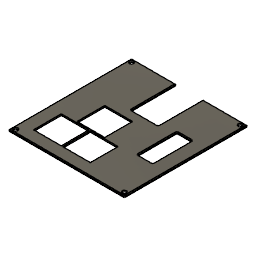
Top (Autodesk Fusion 360 design; units mm, degrees)
part number: 2025-12-11-15-33-41-186
Autodesk Fusion 360 part; units mm, degrees
note: some values were not read from the file. Chosen so that the rebuilt part matches the saved one: a direction; that a step has no effect; which face or edge a step refers to. Set by a fixed rule: which sketch regions a step uses.
sketch "plate-2025-12-11T14_40_51.643Z" plane through (0, 0, 0) normal (0, 0, 1) x (1, 0, 0)
  line L0 (69.2455, 32.444) -> (-10.7545, 32.444)
  line L1 (-10.7545, 32.444) -> (-10.7545, -52.556)
  line L2 (-10.7545, -52.556) -> (69.2455, -52.556)
  line L3 (69.2455, -52.556) -> (69.2455, 32.444)
  line L4 (10.79, 32.444) -> (29.29, 32.444)
  line L5 (64.2455, 27.444) -> (-5.7545, 27.444)
  line L6 (-5.7545, 27.444) -> (-5.7545, -47.556)
  line L7 (-5.7545, -47.556) -> (64.2455, -47.556)
  line L8 (64.2455, -47.556) -> (64.2455, 27.444)
  line L9 (20.04, 63.444) -> (38.54, 63.444)
  line L10 (38.54, 63.444) -> (38.54, 1.444)
  line L11 (38.54, 1.444) -> (20.04, 1.444)
  line L12 (20.04, 1.444) -> (20.04, 63.444)
  circle A0 centre (-8.2545, 29.944) radius 1.45
  circle A1 centre (-8.2545, -50.056) radius 1.45
  circle A2 centre (66.7455, -50.056) radius 1.45
  circle A3 centre (66.7455, 29.944) radius 1.45
  line L13 (8.3105, -5.141) -> (27.3605, -5.141)
  line L14 (27.3605, -5.141) -> (27.3605, -24.191)
  line L15 (27.3605, -24.191) -> (8.3105, -24.191)
  line L16 (8.3105, -24.191) -> (8.3105, -5.141)
  line L17 (18.3405, -25.141) -> (37.3905, -25.141)
  line L18 (37.3905, -25.141) -> (37.3905, -44.191)
  line L19 (37.3905, -44.191) -> (18.3405, -44.191)
  line L20 (18.3405, -44.191) -> (18.3405, -25.141)
  line L21 (-1.7295, -25.146) -> (17.3205, -25.146)
  line L22 (17.3205, -25.146) -> (17.3205, -44.196)
  line L23 (17.3205, -44.196) -> (-1.7295, -44.196)
  line L24 (-1.7295, -44.196) -> (-1.7295, -25.146)
  point P0 (29.29, 32.444)
  dimension "d1" = 80
  dimension "d2" = 85
  dimension "d44" = 75
  dimension "d45" = 70
  dimension "d65" = 2.9
  dimension "d66" = 2.9
  dimension "d67" = 2.9
  dimension "d68" = 2.9
  dimension "d94" = 19.05
  dimension "d95" = 19.05
  dimension "d96" = 19.05
  dimension "d97" = 19.05
  dimension "d98" = 19.05
  dimension "d99" = 19.05
  dimension "d114" = 1.02
  dimension "d116" = 39.12
  dimension "d117" = 10.04
  dimension "d118" = 10.03
  dimension "d119" = 0.95
  dimension "d120" = 70
  dimension "d121" = 5
  dimension "d122" = 5
  dimension "d124" = 25.7945
  dimension "d125" = 2.5
  dimension "d126" = 2.5
  dimension "d127" = 4.025
  dimension "d128" = 2.5
  dimension "d129" = 2.5
  dimension "d130" = 2.5
  dimension "d131" = 2.5
  dimension "d132" = 2.5
  dimension "d133" = 2.5
  dimension "d134" = 18.5
  dimension "d136" = 6.585
  dimension "d138" = 26
  constraint horizontal L0
  constraint perpendicular L0 L1
  constraint parallel L0 L2
  constraint parallel L1 L3
  constraint horizontal L4
  constraint coincident L0 L4.start
  constraint horizontal L5
  constraint perpendicular L5 L6
  constraint parallel L5 L7
  constraint parallel L6 L8
  constraint horizontal L9
  constraint perpendicular L9 L10
  constraint parallel L9 L11
  constraint parallel L10 L12
  constraint coincident P0 L4.end
  constraint horizontal L13
  constraint perpendicular L13 L14
  constraint parallel L13 L15
  constraint parallel L14 L16
  constraint horizontal L17
  constraint perpendicular L17 L18
  constraint parallel L17 L19
  constraint parallel L18 L20
  constraint horizontal L21
  constraint perpendicular L21 L22
  constraint parallel L21 L23
  constraint parallel L22 L24
  measures "d1" distance of L1 L3
  measures "d2" distance of L0 L2
  measures "d44" distance of L5 L7
  measures "d45" distance of L6 L8
  measures "d65" diameter of A0
  measures "d66" diameter of A1
  measures "d67" diameter of A2
  measures "d68" diameter of A3
  measures "d94" distance of L14.end L15.end
  measures "d95" distance of L13.end L14.end
  measures "d96" distance of L18.end L19.end
  measures "d97" distance of L17.end L18.end
  measures "d98" distance of L22.end L23.end
  measures "d99" distance of L21.end L22.end
  measures "d114" distance of L20 L22
  measures "d116" distance of L18 L24
  measures "d117" distance of L16 L24
  measures "d118" distance of L14 L18
  measures "d119" distance of L15 L17
  measures "d120" distance of L6 L8
  measures "d121" distance of L1 L6
  measures "d122" distance of L2 L7
  measures "d124" distance of L6 L12
  measures "d125" distance of L0 A0.centre
  measures "d126" distance of L1 A0.centre
  measures "d127" distance of L6 L24
  measures "d128" distance of L1 A1.centre
  measures "d129" distance of L2 A1.centre
  measures "d130" distance of L3 A2.centre
  measures "d131" distance of L2 A2.centre
  measures "d132" distance of L0 A3.centre
  measures "d133" distance of L3 A3.centre
  measures "d134" distance of L10 L12
  measures "d136" distance of L11 L13
  measures "d138" distance of L5 L11
sketch "Sketch4" plane through (0, 0, 0) normal (0, 0, -1) x (1, 0, 0)
  arc A0 (11.895, 9.31) -> (12.395, 8.81) centre (12.395, 9.31) ccw
  line L0 (11.895, 9.31) -> (11.895, 22.31)
  arc A1 (12.395, 22.81) -> (11.895, 22.31) centre (12.395, 22.31) ccw
  line L1 (12.395, 22.81) -> (25.395, 22.81)
  arc A2 (25.895, 22.31) -> (25.395, 22.81) centre (25.395, 22.31) ccw
  line L2 (25.895, 22.31) -> (25.895, 9.31)
  arc A3 (25.395, 8.81) -> (25.895, 9.31) centre (25.395, 9.31) ccw
  line L3 (25.395, 8.81) -> (12.395, 8.81)
  arc A4 (20.705, 28.36) -> (21.205, 27.86) centre (21.205, 28.36) ccw
  line L4 (20.705, 28.36) -> (20.705, 41.36)
  arc A5 (21.205, 41.86) -> (20.705, 41.36) centre (21.205, 41.36) ccw
  line L5 (21.205, 41.86) -> (34.205, 41.86)
  arc A6 (34.705, 41.36) -> (34.205, 41.86) centre (34.205, 41.36) ccw
  line L6 (34.705, 41.36) -> (34.705, 28.36)
  arc A7 (34.205, 27.86) -> (34.705, 28.36) centre (34.205, 28.36) ccw
  line L7 (34.205, 27.86) -> (21.205, 27.86)
  arc A8 (15.125, 27.86) -> (15.625, 28.36) centre (15.125, 28.36) ccw
  line L8 (15.125, 27.86) -> (2.125, 27.86)
  arc A9 (1.625, 28.36) -> (2.125, 27.86) centre (2.125, 28.36) ccw
  line L9 (1.625, 28.36) -> (1.625, 41.36)
  arc A10 (2.125, 41.86) -> (1.625, 41.36) centre (2.125, 41.36) ccw
  line L10 (2.125, 41.86) -> (15.125, 41.86)
  arc A11 (15.625, 41.36) -> (15.125, 41.86) centre (15.125, 41.36) ccw
  line L11 (15.625, 41.36) -> (15.625, 28.36)
  line L12 (-10.7545, -32.444) -> (20.04, -32.444)
  line L13 (20.04, -32.444) -> (20.04, -1.444)
  line L14 (20.04, -1.444) -> (38.54, -1.444)
  line L15 (38.54, -1.444) -> (38.54, -32.444)
  line L16 (38.54, -32.444) -> (69.2455, -32.444)
  line L17 (69.2455, -32.444) -> (69.2455, 52.556)
  line L18 (69.2455, 52.556) -> (-10.7545, 52.556)
  line L19 (-10.7545, 52.556) -> (-10.7545, -32.444)
  line L20 (59.2455, 22.981) -> (49.0455, 22.981)
  line L21 (49.0455, 22.981) -> (49.0455, -3.919)
  line L22 (49.0455, -3.919) -> (59.2455, -3.919)
  line L23 (59.2455, -3.919) -> (59.2455, 22.981)
  line L24 (64.2455, -27.444) -> (-5.7545, -27.444)
  line L25 (64.2455, 47.556) -> (64.2455, -27.444)
  line L26 (-5.7545, 47.556) -> (64.2455, 47.556)
  dimension "d58" = 10.2
  dimension "d59" = 26.9
  dimension "d60" = 23.525
  dimension "d61" = 5
  dimension "d62" = 24.575
  constraint horizontal L20
  constraint perpendicular L20 L21
  constraint parallel L20 L22
  constraint parallel L21 L23
  measures "d58" distance of L21.end L22.end
  measures "d59" distance of L20.end L21.end
  measures "d60" distance of L22 L24
  measures "d61" distance of L23 L25
  measures "d62" distance of L20 L26
extrude "Extrude7" add sketch "plate-2025-12-11T14_40_51.643Z" sketch "Sketch4" along normal blind 1 contours L0 L1 L2 L3 L4 L5 L6 L7 L8 L10 L12 | L5 L6 L7 L8 L10 L11 L12 | A0 | A1 | A2 | A3 | L13 L14 L15 L16 | L17 L18 L19 L20 | L21 L22 L23 L24 of sketch 2 contours A0 L0 A1 L1 A2 L2 A3 L3 | A4 L4 A5 L5 A6 L6 A7 L7 | A8 L8 A9 L9 A10 L10 A11 L11 | L12 L13 L14 L15 L16 L17 L18 L19 | L20 L21 L22 L23
extrude "Extrude8" cut sketch "plate-2025-12-11T14_40_51.643Z" along normal blind 2 contours A0 | A1 | A2 | A3
fillet "Fillet4" radius 0.5 16 edges at (20.04, 32.444, 0.5) (4.6427, 32.444, 1) (-10.7545, 32.444, 0.5) (20.04, 1.444, 0.5) (20.04, 16.944, 1) (-10.7545, -10.056, 1) (29.2455, -52.556, 1) (29.29, 1.444, 1) (69.2455, -10.056, 1) (38.54, 16.944, 1) (53.8927, 32.444, 1) (-10.7545, -52.556, 0.5) (38.54, 1.444, 0.5) (69.2455, -52.556, 0.5) (69.2455, 32.444, 0.5) (38.54, 32.444, 0.5)
extrude "Extrude9" cut sketch "Sketch4" against normal blind 1 contours L20 L21 L22 L23
fillet "Fillet5" radius 0.5 8 edges at (49.0455, -9.531, 1) (54.1455, 3.919, 1) (59.2455, -9.531, 1) (54.1455, -22.981, 1) (49.0455, 3.919, 0.5) (49.0455, -22.981, 0.5) (59.2455, -22.981, 0.5) (59.2455, 3.919, 0.5)
extrude "Extrude10" cut sketch "plate-2025-12-11T14_40_51.643Z" along normal blind 2 contours L13 L14 L15 L16 | L17 L18 L19 L20 | L21 L22 L23 L24
fillet "Fillet6" [no effect]
